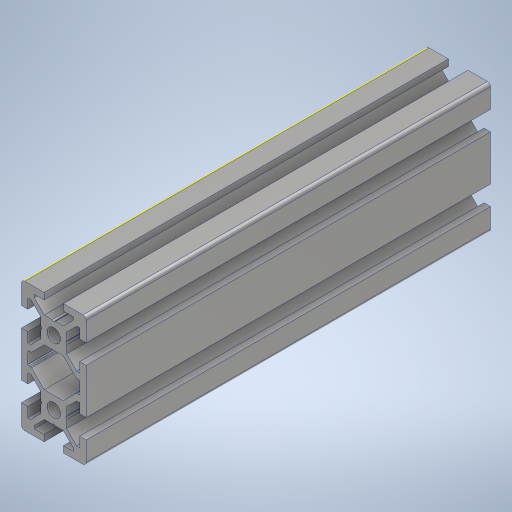
# Autodesk Inventor part: 2040 Z-Rail Brace
Saved by Autodesk Inventor 2024 (Build 280153000, 153)
## iProperties
Category: PARTsolutions
Company: MISUMI
Created: 2024-10-26
Part Number: 2040 Z-Rail Brace
Material: Aluminum 6061
Catalog Web Link: www.cadenas.de
Description: NFS5-2040, NFSB5-2040, HFS5-2040, HFSB5-2040, CAF5-2040, NFSF5-2040, HFSF5-2040, HFSY5-2040-Aluminum Frames -5 Series-2Row Groove 20x40 mm Square -Specified Length
Vendor: MISUMI
Document SubType Name: Modeling
Designer: psAdmin
Manufacturer: MISUMI
Mass: 437.054 g
Surface Area: 1577.39 cm^2
Volume: 161.872 cm^3
Density: 2.7 g/cm^3
Appearance: Aluminum - Flat
PSOL_IDENT_0: {$CADENAS_DATA/23d-libs/misumi/metric/38_al_extrusions_blackets/5/hfs5_2040.prj},633 {VTYP=3D},{NB=H
PSOL_IDENT_1: FS5-2040-500-SC},{LINA=HFS5-2040-500-SC},{NN=NFS5-2040, NFSB5-2040, HFS5-2040, HFSB5-2040, CAF5-2040
PSOL_IDENT_2: , NFSF5-2040, HFSF5-2040, HFSY5-2040},{DATE=08.05.2023 08:39:28},{GEOMDATE=23.09.2021 02:57:03},{VER
PSOL_IDENT_3: SION=},{LINEID=150},{WBVAR=L,ALT1,ALT2,ALT4,ALT5,CP5,DL5,DR5,ALT6,ALT9,ALT10,ALT11,HP6,NHL6,DL6,NHR6
PSOL_IDENT_4: ,DR6,ALT7,ALT8,NH9,AH,BH,CH,DH,EH,NH10,AV,BV,CV,DV,EV,NH11,AP,BP,CP,DP,EP,ALT12,ALT13,Z,NH12,XA,XB,X
PSOL_IDENT_5: C,XD,XE,NH13,YA,YB,YC,YD,YE,ALT16,HP16,DL16,DR16,ALT17,HQ17,JLP,ALT18,HQ18,KLP,ALT20},{WBNUMERIC=L,N
PSOL_IDENT_6: H9,AH,BH,CH,DH,EH,NH10,AV,BV,CV,DV,EV,NH11,AP,BP,CP,DP,EP,NH12,XA,XB,XC,XD,XE,NH13,YA,YB,YC,YD,YE,HQ
PSOL_IDENT_7: 17,JLP,HQ18,KLP}  {NB=HFS5-2040-500-SC},{LINA=HFS5-2040-500-SC},{KT=DUMMY},{PN=HFS5-2040-500-SC},{TP
PSOL_IDENT_8: S=HFS5-2040},{MAT=A6N01SS-T5 Aluminum Alloy},{ST=Clear Anodize},{FRMW=20},{FRMH=40},{FRD=4.2},{L=500
PSOL_IDENT_9: },{MASS=0.88},{SA=324},{LX=1.358x10^4},{LY=5.13x10^4},{ALT1=},{M1=0},{DPL1=0},{DPR1=0},{ALT1PN=},{AL
PSOL_IDENT_10: T2=},{ALT2ALG= '','w/o End Tapping (Insert)','LHP','with LHP (Tapping on the Left (Insert))','RHP','
PSOL_IDENT_11: with RHP (Tapping on the Right (Insert))','HPW','with HPW (Tapping on Both Ends (Insert))' },{M2=0},
PSOL_IDENT_12: {DP2=0},{ALT2PN=},{ALT4=SC},{ALT4ALG= '', 'w/o SC (High Precision Cut)', 'SC', 'with SC (High Precis
PSOL_IDENT_13: ion Cut)' },{ALT4PN=-SC},{ALT5=},{ALT5ALG= '','w/o 45 Degree Cut','1','with 45 Degree Cut' },{CP5=},
PSOL_IDENT_14: {CP5ALG= '','N/A' },{DL5=},{DL5ALG= '','N/A' },{DR5=},{DR5ALG= '','N/A' },{FRMLALT5=0},{FRMRALT5=0},
PSOL_IDENT_15: {ALT5PN=},{ALT6=},{ALT6ALG= '','w/o Fastening Location Wrench Access Hole Alterations','1','with Fas
PSOL_IDENT_16: tening Location Wrench Access Hole Alterations' },{ALT9=},{ALT9ALG= '','w/o Location Specified Wrenc
PSOL_IDENT_17: h Access Hole Alteratons (Horizontal)','1','with Location Specified Wrench Access Hole Alteratons (H
PSOL_IDENT_18: orizontal)' },{ALT10=},{ALT10ALG= '','w/o Location Specified Wrench Access Hole Alteratons (Vertical
PSOL_IDENT_19: )','1','with Location Specified Wrench Access Hole Alteratons (Vertical)' },{ALT11=},{ALT11ALG= '','
PSOL_IDENT_20: w/o Location Specified Wrench Access Hole Alteratons (Crisscross)','1','with Location Specified Wren
PSOL_IDENT_21: ch Access Hole Alteratons (Crisscross)' },{HP6=},{HP6ALG= '','N/A' },{NHL6=},{NHL6ALG= '','N/A' },{D
PSOL_IDENT_22: L6=},{DL6ALG= '','N/A' },{NHR6=},{NHR6ALG= '','N/A' },{DR6=},{DR6ALG= '','N/A' },{HL6=0},{HL6D=0},{H
PSOL_IDENT_23: R6=0},{HR6D=0},{J6=0},{J6D=0},{K6=0},{K6D=0},{DD6=0.00},{DD6ALG=0},{ALT7=},{ALT7ALG= '','N/A' },{ALT
PSOL_IDENT_24: 8=},{ALT8ALG= '','N/A' },{ALT678PN=},{NH9=0},{NH9MAX=5},{NH9ALG=[0]},{AH=0.0},{AHMIN=7},{AHMAX=495},
PSOL_IDENT_25: {AHALG=[0]},{BH=0.0},{BHMIN=2},{BHMAX=497},{BHALG=[0]},{CH=0.0},{CHMIN=2},{CHMAX=499},{CHALG=[0]},{D
PSOL_IDENT_26: H=0.0},{DHMIN=2},{DHMAX=501},{DHALG=[0]},{EH=0.0},{EHMIN=2},{EHMAX=493},{EHALG=[0]},{NH10=0},{NH10MA
PSOL_IDENT_27: X=5},{NH10ALG=[0]},{AV=0.0},{AVMIN=7},{AVMAX=495},{AVALG=[0]},{BV=0.0},{BVMIN=2},{BVMAX=497},{BVALG=
PSOL_IDENT_28: [0]},{CV=0.0},{CVMIN=2},{CVMAX=499},{CVALG=[0]},{DV=0.0},{DVMIN=2},{DVMAX=501},{DVALG=[0]},{EV=0.0},
PSOL_IDENT_29: {EVMIN=2},{EVMAX=493},{EVALG=[0]},{NH11=0},{NH11MAX=5},{NH11ALG=[0]},{AP=0.0},{APMIN=7},{APMAX=495},
PSOL_IDENT_30: {APALG=[0]},{BP=0.0},{BPMIN=2},{BPMAX=497},{BPALG=[0]},{CP=0.0},{CPMIN=2},{CPMAX=499},{CPALG=[0]},{D
PSOL_IDENT_31: P=0.0},{DPMIN=2},{DPMAX=501},{DPALG=[0]},{EP=0.0},{EPMIN=2},{EPMAX=493},{EPALG=[0]},{ALT9PN=},{ALT10
PSOL_IDENT_32: PN=},{ALT11PN=},{ALT91011PN=},{ALT12=},{ALT12ALG= '','w/o Counterbore Hole in Specified Position (Ve
PSOL_IDENT_33: rtical)','1','with Counterbore Hole in Specified Position (Vertical)' },{ALT13=},{ALT13ALG= '','w/o
PSOL_IDENT_34: Counterbore Hole in Specified Position (Horizontal)','1','with Counterbore Hole in Specified Positio
PSOL_IDENT_35: n (Horizontal)' },{Z=},{ZALG= '','N/A' },{DD12=0.0},{DD112=0.0},{NH12=0},{NH12MAX=5},{NH12ALG=[0]},{
PSOL_IDENT_36: XA=0.0},{XAMIN=7},{XAMAX=495},{XAALG=[0]},{XB=0.0},{XBMIN=2},{XBMAX=497},{XBALG=[0]},{XC=0.0},{XCMIN=
PSOL_IDENT_37: 2},{XCMAX=499},{XCALG=[0]},{XD=0.0},{XDMIN=2},{XDMAX=501},{XDALG=[0]},{XE=0.0},{XEMIN=2},{XEMAX=493}
PSOL_IDENT_38: ,{XEALG=[0]},{NH13=0},{NH13MAX=5},{NH13ALG=[0]},{YA=0.0},{YAMIN=7},{YAMAX=495},{YAALG=[0]},{YB=0.0},
PSOL_IDENT_39: {YBMIN=2},{YBMAX=497},{YBALG=[0]},{YC=0.0},{YCMIN=2},{YCMAX=499},{YCALG=[0]},{YD=0.0},{YDMIN=2},{YDM
PSOL_IDENT_40: AX=501},{YDALG=[0]},{YE=0.0},{YEMIN=2},{YEMAX=493},{YEALG=[0]},{ALT12PN=},{ALT13PN=},{ALT1213PN=},{A
PSOL_IDENT_41: LT16=},{ALT16ALG= '','w/o M Type Hole Alteration','1','with M Type Hole Alteration' },{HP16=},{HP16A
PSOL_IDENT_42: LG= '','N/A' },{DL16=},{DL16ALG= '','N/A' },{DR16=},{DR16ALG= '','N/A' },{H116=0},{D16=0.0},{ALT16PN=
PSOL_IDENT_43: },{ALT17=},{ALT17ALG= '','w/o L Type Hole Alteration (Top)','1','with L Type Hole Alteration (Top)'
PSOL_IDENT_44: },{HQ17=0},{HQ17ALG=0},{JLP=0},{JLPMIN=4.9},{JLPMAX=0},{JLPALG=[0]},{L17=0},{D17=0.0},{ALT18=},{ALT1
PSOL_IDENT_45: 8ALG= '','w/o L Type Hole Alteration (Bottom)','1','with L Type Hole Alteration (Bottom)' },{HQ18=0}
PSOL_IDENT_46: ,{HQ18ALG=0},{KLP=0},{KLPMIN=4.9},{KLPMAX=0},{KLPALG=[0]},{L18=0},{D18=0.0},{ALT1718PN=},{ALT20=},{A
PSOL_IDENT_47: LT20PN=},{ERRORALT01=OK},{ERRORALT02=OK},{ERRORALT05=OK},{ERRORALT06091=OK},{ERRORALT06092=OK},{ERRO
PSOL_IDENT_48: RALT06093=OK},{ERRORALT06094=OK},{ERRORALT06101=OK},{ERRORALT06102=OK},{ERRORALT06103=OK},{ERRORALT0
PSOL_IDENT_49: 6104=OK},{ERRORALT06111=OK},{ERRORALT06112=OK},{ERRORALT06113=OK},{ERRORALT06114=OK},{ERRORALT06121=
PSOL_IDENT_50: OK},{ERRORALT06122=OK},{ERRORALT06123=OK},{ERRORALT06124=OK},{ERRORALT06131=OK},{ERRORALT06132=OK},{
PSOL_IDENT_51: ERRORALT06133=OK},{ERRORALT06134=OK},{ERRORALT0616=OK},{ERRORALT06171=OK},{ERRORALT06172=OK},{ERRORA
PSOL_IDENT_52: LT06173=OK},{ERRORALT06181=OK},{ERRORALT06182=OK},{ERRORALT06183=OK},{ERRORALT0911=OK},{ERRORALT0913=
PSOL_IDENT_53: OK},{ERRORALT0916=OK},{ERRORALT0917=OK},{ERRORALT0918=OK},{ERRORALT1011=OK},{ERRORALT1012=OK},{ERROR
PSOL_IDENT_54: ALT1016=OK},{ERRORALT1017=OK},{ERRORALT1018=OK},{ERRORALT1112=OK},{ERRORALT1113=OK},{ERRORALT1116=OK
PSOL_IDENT_55: },{ERRORALT1117=OK},{ERRORALT1118=OK},{ERRORALT1216=OK},{ERRORALT1217=OK},{ERRORALT1218=OK},{ERRORAL
PSOL_IDENT_56: T1316=OK},{ERRORALT1317=OK},{ERRORALT1318=OK},{ERRORALT1617=OK},{ERRORALT1618=OK},{ERRORPN=},{TFW=0}
PSOL_IDENT_57: ,{COLOR=}
NB: HFS5-2040-500-SC
NN: NFS5-2040, NFSB5-2040, HFS5-2040, HFSB5-2040, CAF5-2040, NFSF5-2040, HFSF5-2040, HFSY5-2040
NT: Aluminum Frames -5 Series-2Row Groove 20x40 mm Square -Specified Length
NBSYN: $PN.
LINA: HFS5-2040-500-SC
CATALOG: Misumi
PN: HFS5-2040-500-SC
TPS: HFS5-2040
MAT: A6N01SS-T5 Aluminum Alloy
ST: Clear Anodize
L: 500
MASS: 0.88
SA: 324
LX: 1.358x10^4
LY: 5.13x10^4
ALT1: w/o End Tapping
M1: 0
DPL1: 0
DPR1: 0
ALT2: w/o End Tapping (Insert)
M2: 0
DP2: 0
ALT4: with SC (High Precision Cut)
ALT5: w/o 45 Degree Cut
CP5: N/A
DL5: N/A
DR5: N/A
ALT6: w/o Fastening Location Wrench Access Hole Alterations
ALT9: w/o Location Specified Wrench Access Hole Alteratons (Horizontal)
ALT10: w/o Location Specified Wrench Access Hole Alteratons (Vertical)
ALT11: w/o Location Specified Wrench Access Hole Alteratons (Crisscross)
HP6: N/A
NHL6: N/A
DL6: N/A
NHR6: N/A
DR6: N/A
HL6D: 0
HR6D: 0
J6D: 0
K6D: 0
DD6: 0
ALT7: N/A
ALT8: N/A
NH9: 0
AH: 0
BH: 0
CH: 0
DH: 0
EH: 0
NH10: 0
AV: 0
BV: 0
CV: 0
DV: 0
EV: 0
NH11: 0
AP: 0
BP: 0
CP: 0
DP: 0
EP: 0
ALT12: w/o Counterbore Hole in Specified Position (Vertical)
ALT13: w/o Counterbore Hole in Specified Position (Horizontal)
Z: N/A
DD12: 0
DD112: 0
NH12: 0
XA: 0
XB: 0
XC: 0
XD: 0
XE: 0
NH13: 0
YA: 0
YB: 0
YC: 0
YD: 0
YE: 0
ALT16: w/o M Type Hole Alteration
HP16: N/A
DL16: N/A
DR16: N/A
H116: 0
D16: 0
ALT17: w/o L Type Hole Alteration (Top)
HQ17: 0
JLP: 0
D17: 0
ALT18: w/o L Type Hole Alteration (Bottom)
HQ18: 0
KLP: 0
D18: 0
ALT20: w/o CW (End Face C Chamfering)
SUPPLIER: MISUMI
ARTICLENO: HFS5-2040-500-SC
BOMINFO: HFS5-2040-500-SC
CREATOR: CADENAS GmbH
Title: HFS5-2040-500-SC
Author: Cadenas PARTsolutions
Comments: Aluminum Frames -5 Series-2Row Groove 20x40 mm Square -Specified Length
Autodesk Inventor part; units mm, degrees
sketch "Sketch_1" plane through (0, 0, 0) normal (0, 0, 1) x (1, 0, 0)
  line L0 (-10, -7) -> (-8, -7)
  line L1 (-8, -7) -> (-8, -4)
  line L2 (-8, -4) -> (-7.0607, -4)
  line L3 (-7.0607, -4) -> (-4, -7.0607)
  line L4 (-4, -7.0607) -> (-4, -9.4804)
  line L5 (-4, -9.4804) -> (-3.7, -10)
  line L6 (-3.7, -10) -> (-4, -10.5196)
  line L7 (-4, -10.5196) -> (-4, -12.9393)
  line L8 (-4, -12.9393) -> (-7.0607, -16)
  line L9 (-7.0607, -16) -> (-8, -16)
  line L10 (-8, -16) -> (-8, -13)
  line L11 (-8, -13) -> (-10, -13)
  line L12 (-10, -13) -> (-10, -19)
  arc A0 (-10, -19) -> (-9, -20) centre (-9, -19) ccw
  line L13 (-9, -20) -> (-3, -20)
  line L14 (-3, -20) -> (-3, -18)
  line L15 (-3, -18) -> (-6, -18)
  line L16 (-6, -18) -> (-6, -17.0607)
  line L17 (-6, -17.0607) -> (-2.9393, -14)
  line L18 (-2.9393, -14) -> (-0.5196, -14)
  line L19 (-0.5196, -14) -> (0, -13.7)
  line L20 (0, -13.7) -> (0.5196, -14)
  line L21 (0.5196, -14) -> (2.9393, -14)
  line L22 (2.9393, -14) -> (6, -17.0607)
  line L23 (6, -17.0607) -> (6, -18)
  line L24 (6, -18) -> (3, -18)
  line L25 (3, -18) -> (3, -20)
  line L26 (3, -20) -> (9, -20)
  arc A1 (9, -20) -> (10, -19) centre (9, -19) ccw
  line L27 (10, -19) -> (10, -13)
  line L28 (10, -13) -> (8, -13)
  line L29 (8, -13) -> (8, -16)
  line L30 (8, -16) -> (7.0607, -16)
  line L31 (7.0607, -16) -> (4, -12.9393)
  line L32 (4, -12.9393) -> (4, -10.5196)
  line L33 (4, -10.5196) -> (3.7, -10)
  line L34 (3.7, -10) -> (4, -9.4804)
  line L35 (4, -9.4804) -> (4, -7.0607)
  line L36 (4, -7.0607) -> (7.0607, -4)
  line L37 (7.0607, -4) -> (8, -4)
  line L38 (8, -4) -> (8, -7)
  line L39 (8, -7) -> (10, -7)
  line L40 (10, -7) -> (10, 7)
  line L41 (10, 7) -> (8, 7)
  line L42 (8, 7) -> (8, 4)
  line L43 (8, 4) -> (7.0607, 4)
  line L44 (7.0607, 4) -> (4, 7.0607)
  line L45 (4, 7.0607) -> (4, 9.4804)
  line L46 (4, 9.4804) -> (3.7, 10)
  line L47 (3.7, 10) -> (4, 10.5196)
  line L48 (4, 10.5196) -> (4, 12.9393)
  line L49 (4, 12.9393) -> (7.0607, 16)
  line L50 (7.0607, 16) -> (8, 16)
  line L51 (8, 16) -> (8, 13)
  line L52 (8, 13) -> (10, 13)
  line L53 (10, 13) -> (10, 19)
  arc A2 (10, 19) -> (9, 20) centre (9, 19) ccw
  line L54 (9, 20) -> (3, 20)
  line L55 (3, 20) -> (3, 18)
  line L56 (3, 18) -> (6, 18)
  line L57 (6, 18) -> (6, 17.0607)
  line L58 (6, 17.0607) -> (2.9393, 14)
  line L59 (2.9393, 14) -> (0.5196, 14)
  line L60 (0.5196, 14) -> (0, 13.7)
  line L61 (0, 13.7) -> (-0.5196, 14)
  line L62 (-0.5196, 14) -> (-2.9393, 14)
  line L63 (-2.9393, 14) -> (-6, 17.0607)
  line L64 (-6, 17.0607) -> (-6, 18)
  line L65 (-6, 18) -> (-3, 18)
  line L66 (-3, 18) -> (-3, 20)
  line L67 (-3, 20) -> (-9, 20)
  arc A3 (-9, 20) -> (-10, 19) centre (-9, 19) ccw
  line L68 (-10, 19) -> (-10, 13)
  line L69 (-10, 13) -> (-8, 13)
  line L70 (-8, 13) -> (-8, 16)
  line L71 (-8, 16) -> (-7.0607, 16)
  line L72 (-7.0607, 16) -> (-4, 12.9393)
  line L73 (-4, 12.9393) -> (-4, 10.5196)
  line L74 (-4, 10.5196) -> (-3.7, 10)
  line L75 (-3.7, 10) -> (-4, 9.4804)
  line L76 (-4, 9.4804) -> (-4, 7.0607)
  line L77 (-4, 7.0607) -> (-7.0607, 4)
  line L78 (-7.0607, 4) -> (-8, 4)
  line L79 (-8, 4) -> (-8, 7)
  line L80 (-8, 7) -> (-10, 7)
  line L81 (-10, 7) -> (-10, -7)
  line L82 (-8, 1.7) -> (-8, -1.7)
  arc A4 (-8, -1.7) -> (-7.7, -2) centre (-7.7, -1.7) ccw
  line L83 (-7.7, -2) -> (-7.0636, -2)
  arc A5 (-6.8515, -2.0879) -> (-7.0636, -2) centre (-7.0636, -2.3) ccw
  line L84 (-6.8515, -2.0879) -> (-2.9393, -6)
  line L85 (-2.9393, -6) -> (2.9393, -6)
  line L86 (2.9393, -6) -> (6.8515, -2.0879)
  arc A6 (7.0636, -2) -> (6.8515, -2.0879) centre (7.0636, -2.3) ccw
  line L87 (7.0636, -2) -> (7.7, -2)
  arc A7 (7.7, -2) -> (8, -1.7) centre (7.7, -1.7) ccw
  line L88 (8, -1.7) -> (8, 1.7)
  arc A8 (8, 1.7) -> (7.7, 2) centre (7.7, 1.7) ccw
  line L89 (7.7, 2) -> (7.0636, 2)
  arc A9 (6.8515, 2.0879) -> (7.0636, 2) centre (7.0636, 2.3) ccw
  line L90 (6.8515, 2.0879) -> (2.9393, 6)
  line L91 (2.9393, 6) -> (-2.9393, 6)
  line L92 (-2.9393, 6) -> (-6.8515, 2.0879)
  arc A10 (-7.0636, 2) -> (-6.8515, 2.0879) centre (-7.0636, 2.3) ccw
  line L93 (-7.0636, 2) -> (-7.7, 2)
  arc A11 (-7.7, 2) -> (-8, 1.7) centre (-7.7, 1.7) ccw
  constraints: 188 end point, 24 point on circle, 12 centre point
extrude "Extrusion1" add sketch "Sketch_1" along normal mid plane 125
sketch "Sketch2" plane through (0, 0, 62.5) normal (0, 0, 1) x (-1, 0, 0)
  point P0 (0, 10)
hole "Hole1" at (0, -10, 62.5) direction (0, 0, -1) diameter 4.134 end through all thread size "M5x0.8" class "6H" standard "ANSI Metric M Profile"
pattern_linear "Rectangular Pattern1" count 2 spacing 20 along (0, 1, 0) of "Hole1"
ref_plane "C1_XY" through (0, 0, 0) normal (0, 0, 1) x (1, 0, 0)
ref_plane "C1_YZ" through (0, 0, 0) normal (1, 0, 0) x (0, 1, 0)
ref_plane "C1_ZX" through (0, 0, 0) normal (0, 1, 0) x (0, 0, 1)
mirror "Mirror1" about plane through (0, 0, 0) normal (0, 0, 1) of "Hole1", "Rectangular Pattern1"
body "Solid1"
